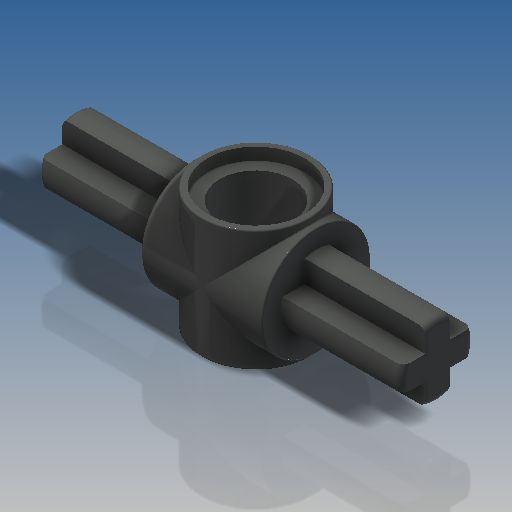
# Autodesk Inventor part: 27940-DkBluishGray
Saved by Autodesk Inventor 2019.4 (Build 234330000, 330)
## iProperties
Created: 2016-01-22
Part Number: 27940-DkBluishGray
Material: ABS Plastic
Document SubType Name: Modeling
Designer: D. Kohfeld
Density: 1.06 g/cm^3
Appearance: DkBluishGray
Mass: 0.460947 g
Surface Area: 6.9483 cm^2
Volume: 0.434855 cm^3
Author: D. Kohfeld
Autodesk Inventor part; units mm, degrees
ref_plane "YZ Plane" through (0, 0, 0) normal (1, 0, 0) x (0, 1, 0)
ref_plane "XZ Plane" through (0, 0, 0) normal (0, 1, 0) x (-1, 0, 0)
ref_plane "XY Plane" through (0, 0, 0) normal (0, 0, 1) x (1, 0, 0)
sketch "Sketch2" plane through (0, 0, 0) normal (0, 1, 0) x (-1, 0, 0)
  circle A0 centre (0, 0) radius 3.6
  circle A1 centre (0, 0) radius 3.2
  circle A2 centre (0, 0) radius 2.4
  line L0 (0, 0) -> (-4, 0)
  line L1 (-4, 0) -> (-4, 3.6)
  line L2 (-4, 3.6) -> (0, 3.6)
  line L3 (0, 3.6) -> (0, 0)
  dimension "d0" = 4.8
  dimension "d1" = 6.4
  dimension "d2" = 7.2
  dimension "d3" = 4
  dimension "d4" = 7.2
  constraints: 8 end point, 3 centre point, 3 coincident, 2 parallel, 1 horizontal, 1 perpendicular
  measures "d0" diameter of A2
  measures "d1" diameter of A1
  measures "d2" diameter of A0
  measures "d3" distance between parallel lines of L3 L1
  measures "d4" diameter of L2 L0
extrude "Extrusion1" add sketch "Sketch2" along normal mid plane 8 contours A0 L0 A1 L3 | L3 A1 L0 A0 | L3 A2 L0 A1 | A1 L0 A2 L3 | L3 L0 A2 | A2 L0 L3
revolve "Revolution1" add sketch "Sketch2" angle 360 about axis through (0, 0, 0) along (1, 0, 0) picked at (-3.4098, 0.5044) picked at (-2.9066, 0.2374) picked at (-0.178, 1.5799) contours L3 A1 L0 A0 | A0 L0 L1 L2 | L3 A2 L0 A1 | L3 L0 A2
sketch "Sketch3" plane through (4, 0, 0) normal (1, 0, 0) x (0, 0, -1)
  circle A0 centre (0, 0) radius 3.6 projected
  circle A1 centre (0, 0) radius 2.4 construction
  line L0 (-0.8, 2.2627) -> (-0.8, 0.8)
  line L1 (-0.8, 0.8) -> (-2.2627, 0.8)
  line L2 (-2.2627, -0.8) -> (-0.8, -0.8)
  line L3 (-0.8, -0.8) -> (-0.8, -2.2627)
  line L4 (0.8, -2.2627) -> (0.8, -0.8)
  line L5 (0.8, -0.8) -> (2.2627, -0.8)
  line L6 (2.2627, 0.8) -> (0.8, 0.8)
  line L7 (0.8, 0.8) -> (0.8, 2.2627)
  arc A2 (0.8, 2.2627) -> (-0.8, 2.2627) centre (0, 0) ccw
  arc A3 (-2.2627, 0.8) -> (-2.2627, -0.8) centre (0, 0) ccw
  arc A4 (-0.8, -2.2627) -> (0.8, -2.2627) centre (0, 0) ccw
  arc A5 (2.2627, -0.8) -> (2.2627, 0.8) centre (0, 0) ccw
  dimension "d13" = 4.8
  dimension "d12" = 1.6
  constraints: 16 end point, 8 point on circle, 7 equal length, 4 centre point, 4 horizontal, 4 vertical, 1 coincident, 14 other
  measures "d12" distance between parallel lines of L7 L0
extrude "Extrusion4" add sketch "Sketch3" along normal blind 8 contours A2 L7 L6 A5 L5 L4 A4 L3 L2 A3 L1 L0
pattern_circular "Circular Pattern1" count 2 over 360 about axis through (0, 0, 0) along (0, 1, 0) of "Revolution1", "Extrusion4"
extrude "Extrusion2" cut sketch "Sketch2" along normal through all both and the other way through all contours L3 A2 L0 A1 | A1 L0 A2 L3 | L3 L0 A2 | A2 L0 L3
extrude "Extrusion3" add sketch "Sketch2" along normal mid plane 6.4 contours L3 A2 L0 A1 | A1 L0 A2 L3
fillet "Fillet1" radius 0.1 4 edges at (3.6, 4, 0) (3.6, -4, 0) (4, 0, -3.6) (-4, 0, 3.6)
fillet "Fillet1" radius 0.4 8 edges at (12, 0, 2.4) (12, 2.4, 0) (12, 0, -2.4) (12, -2.4, 0) (-12, 0, 2.4) (-12, 2.4, 0) (-12, -2.4, 0) (-12, 0, -2.4)
equation "\"d0\" = tpd"
equation "\"d1\" = tsd"
equation "\"d2\" = tlad"
equation "\"d4\" = d2"
equation "\"d5\" = lu"
equation "\"d13\" = kd"
equation "\"d12\" = axlet"
equation "\"d14\" = lu"
equation "\"d8\" = lu"
equation "\"d10\" = lu - 2 * tsl"
equation "\"d16\" = lf"
equation "\"d17\" = tf"
equation "\"tpd\" = 4.8"
equation "\"tsd\" = 6.4"
equation "\"tlad\" = 7.2"
equation "\"lu\" = 8"
equation "\"kd\" = 4.8"
equation "\"axlet\" = 1.6"
equation "\"tsl\" = 0.8"
equation "\"lf\" = 0.1"
equation "\"tf\" = 0.4"
body "Solid1"
